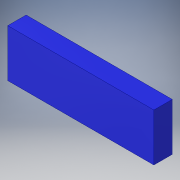
# Autodesk Inventor part: Battery
Saved by Autodesk Inventor 2019 (Build 230136000, 136)
## iProperties
Created: 2019-02-21
Part Number: Battery
Material: Generic
Document SubType Name: Modeling
Designer: varun
Density: 1 g/cm^3
Appearance: Blue - Wall Paint - Glossy
Author: varun
Autodesk Inventor part; units mm, degrees
ref_plane "YZ Plane" through (0, 0, 0) normal (1, 0, 0) x (0, 1, 0)
ref_plane "XZ Plane" through (0, 0, 0) normal (0, 1, 0) x (-1, 0, 0)
ref_plane "XY Plane" through (0, 0, 0) normal (0, 0, 1) x (1, 0, 0)
sketch "Sketch1" plane through (0, 0, 0) normal (0, 0, 1) x (1, 0, 0)
  line L0 (-67.5, 22) -> (67.5, 22)
  line L1 (67.5, 22) -> (67.5, -22)
  line L2 (67.5, -22) -> (-67.5, -22)
  line L3 (-67.5, -22) -> (-67.5, 22)
  line L4 (-67.5, 22) -> (67.5, -22) construction
  line L5 (67.5, 22) -> (-67.5, -22) construction
  point P0 (0, 0)
  dimension "d0" = 135
  dimension "d1" = 44
  constraints: 12 end point, 2 midpoint, 2 parallel, 1 horizontal, 1 perpendicular
  measures "d0" distance of L1.end L2.end
  measures "d1" distance of L0.end L1.end
extrude "Extrusion1" add sketch "Sketch1" along normal blind 17
body "Solid1"
